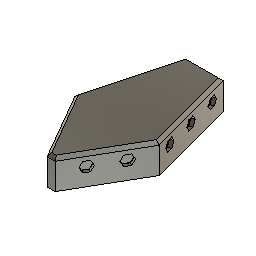
wedge_15deg_2mm (Autodesk Fusion 360 design; units mm, degrees)
Autodesk Fusion 360 part; units mm, degrees
sketch "case_bottom" plane through (0, 0, 0) normal (0, 0, 1) x (1, 0, 0)
  line L0 (-130.2878, -97.5223) -> (-16.5068, -128.0098)
  line L1 (-109.1239, -18.5374) -> (-130.2878, -97.5223)
  line L2 (-16.5068, -128.0098) -> (-3.6943, -109.7118)
  line L3 (-86.9858, -11.6525) -> (-109.1239, -18.5374)
  line L4 (-47.4404, -17.0197) -> (-47.5261, -16.9782)
  line L5 (-47.5261, -16.9782) -> (-66.0896, -12.0041)
  line L6 (-10.9673, -34.7188) -> (-47.4404, -17.0197)
  line L7 (-3.6943, -109.7118) -> (-22.3971, -77.3753)
  line L8 (-22.3971, -77.3753) -> (-10.9673, -34.7188)
  line L9 (-66.0896, -12.0041) -> (-86.9858, -11.6525)
  line L10 (-111.5937, -16.1638) -> (-133.962, -99.6436)
  line L11 (-133.962, -99.6436) -> (-15.2542, -131.4513)
  line L12 (-46.4735, -14.1544) -> (-65.6699, -9.0107)
  line L13 (-65.6699, -9.0107) -> (-87.4169, -8.6449)
  line L14 (-15.2542, -131.4513) -> (-0.1397, -109.8656)
  line L15 (-19.1773, -76.9502) -> (-7.4281, -33.1016)
  line L16 (-0.1397, -109.8656) -> (-19.1773, -76.9502)
  line L17 (-87.4169, -8.6449) -> (-111.5937, -16.1638)
  line L18 (-7.4281, -33.1016) -> (-46.4735, -14.1544)
  line L19 (-65.9217, -10.8067) -> (-87.1583, -10.4495)
  line L20 (-110.1118, -17.588) -> (-131.7575, -98.3709)
  line L21 (-9.5516, -34.0719) -> (-47.1051, -15.8486)
  line L22 (-16.0057, -129.3864) -> (-2.2725, -109.7733)
  line L23 (-47.1051, -15.8486) -> (-65.9217, -10.8067)
  line L24 (-87.1583, -10.4495) -> (-110.1118, -17.588)
  line L25 (-2.2725, -109.7733) -> (-21.1092, -77.2053)
  line L26 (-21.1092, -77.2053) -> (-9.5516, -34.0719)
  line L27 (-131.7575, -98.3709) -> (-16.0057, -129.3864)
  line L28 (-65.8378, -10.208) -> (-87.2445, -9.8479)
  line L29 (-132.4923, -98.7951) -> (-15.7552, -130.0747)
  line L30 (-110.6057, -17.1133) -> (-132.4923, -98.7951)
  line L31 (-46.6545, -15.4003) -> (-46.8946, -15.2839)
  line L32 (-1.5615, -109.8041) -> (-20.4652, -77.1202)
  line L33 (-20.4652, -77.1202) -> (-8.8438, -33.7485)
  line L34 (-15.7552, -130.0747) -> (-1.5615, -109.8041)
  line L35 (-46.8946, -15.2839) -> (-65.8378, -10.208)
  line L36 (-87.2445, -9.8479) -> (-110.6057, -17.1133)
  line L37 (-8.8438, -33.7485) -> (-46.6545, -15.4003)
  circle A0 centre (-88.6378, -32.8795) radius 2.2
  circle A1 centre (-98.4729, -69.5847) radius 2.2
  circle A2 centre (-38.4097, -46.3381) radius 2.2
  circle A3 centre (-34.1664, -92.8451) radius 2.2
  line L38 (-91.0167, -86.1903) -> (-122.8923, -77.6493)
  line L39 (-95.6755, -103.577) -> (-91.0167, -86.1903)
  line L40 (-127.551, -95.0359) -> (-95.6755, -103.577)
  line L41 (-122.8923, -77.6493) -> (-127.551, -95.0359)
  line L42 (-91.5925, -101.9586) -> (-93.1066, -107.6092)
  line L43 (-84.6064, -109.8868) -> (-83.0923, -104.2362)
  line L44 (-83.0923, -104.2362) -> (-91.5925, -101.9586)
  line L45 (-73.6279, -111.4154) -> (-72.7221, -108.0346)
  line L46 (-81.4154, -105.7053) -> (-82.3213, -109.086)
  line L47 (-82.3213, -109.086) -> (-73.6279, -111.4154)
  line L48 (-72.7221, -108.0346) -> (-81.4154, -105.7053)
  line L49 (-12.163, -97.5479) -> (-17.663, -88.0216)
  line L50 (-20.0438, -102.0979) -> (-12.163, -97.5479)
  line L51 (-25.5438, -92.5716) -> (-20.0438, -102.0979)
  line L52 (-17.663, -88.0216) -> (-25.5438, -92.5716)
  line L53 (-96.4921, -72.2377) -> (-98.7956, -80.8345)
  line L54 (-98.7956, -80.8345) -> (-90.4886, -83.0603)
  line L55 (-90.4886, -83.0603) -> (-88.1851, -74.4636)
  line L56 (-88.1851, -74.4636) -> (-96.4921, -72.2377)
  line L57 (1.8603, -131.9251) -> (1.8603, -9.9671)
  line L58 (88.327, -109.8868) -> (86.8129, -104.2362)
  line L59 (137.6826, -99.6436) -> (18.9748, -131.4513)
  line L60 (69.3905, -9.0107) -> (91.1375, -8.6449)
  line L61 (90.7065, -11.6525) -> (112.8445, -18.5374)
  line L62 (90.9651, -9.8479) -> (114.3264, -17.1133)
  line L63 (134.0084, -97.5223) -> (20.2274, -128.0098)
  line L64 (90.8789, -10.4495) -> (113.8324, -17.588)
  line L65 (29.2644, -92.5716) -> (23.7644, -102.0979)
  line L66 (86.8129, -104.2362) -> (95.3131, -101.9586)
  line L67 (21.3836, -88.0216) -> (29.2644, -92.5716)
  line L68 (131.2716, -95.0359) -> (99.3961, -103.577)
  line L69 (50.6152, -15.2839) -> (69.5584, -10.208)
  line L70 (15.8836, -97.5479) -> (21.3836, -88.0216)
  line L71 (91.1375, -8.6449) -> (115.3143, -16.1638)
  line L72 (18.9748, -131.4513) -> (3.8603, -109.8656)
  line L73 (14.6879, -34.7188) -> (51.161, -17.0197)
  line L74 (94.7373, -86.1903) -> (126.6129, -77.6493)
  line L75 (115.3143, -16.1638) -> (137.6826, -99.6436)
  line L76 (5.2822, -109.8041) -> (24.1859, -77.1202)
  line L77 (95.3131, -101.9586) -> (96.8272, -107.6092)
  line L78 (7.4149, -109.7118) -> (26.1177, -77.3753)
  line L79 (99.3961, -103.577) -> (94.7373, -86.1903)
  line L80 (77.3486, -111.4154) -> (76.4427, -108.0346)
  line L81 (69.8103, -12.0041) -> (90.7065, -11.6525)
  line L82 (113.8324, -17.588) -> (135.4781, -98.3709)
  line L83 (19.7263, -129.3864) -> (5.9931, -109.7733)
  line L84 (69.5584, -10.208) -> (90.9651, -9.8479)
  line L85 (91.9058, -74.4636) -> (100.2127, -72.2377)
  line L86 (11.1488, -33.1016) -> (50.1942, -14.1544)
  line L87 (114.3264, -17.1133) -> (136.213, -98.7951)
  line L88 (5.9931, -109.7733) -> (24.8298, -77.2053)
  circle A4 centre (42.1303, -46.3381) radius 2.2
  line L89 (102.5162, -80.8345) -> (94.2092, -83.0603)
  line L90 (85.136, -105.7053) -> (86.0419, -109.086)
  line L91 (69.6424, -10.8067) -> (90.8789, -10.4495)
  line L92 (50.3752, -15.4003) -> (50.6152, -15.2839)
  line L93 (50.1942, -14.1544) -> (69.3905, -9.0107)
  line L94 (22.898, -76.9502) -> (11.1488, -33.1016)
  line L95 (51.161, -17.0197) -> (51.2467, -16.9782)
  line L96 (94.2092, -83.0603) -> (91.9058, -74.4636)
  line L97 (13.2722, -34.0719) -> (50.8257, -15.8486)
  line L98 (112.8445, -18.5374) -> (134.0084, -97.5223)
  line L99 (100.2127, -72.2377) -> (102.5162, -80.8345)
  line L100 (19.4758, -130.0747) -> (5.2822, -109.8041)
  circle A5 centre (102.1935, -69.5847) radius 2.2
  line L101 (50.8257, -15.8486) -> (69.6424, -10.8067)
  circle A6 centre (37.887, -92.8451) radius 2.2
  line L102 (24.1859, -77.1202) -> (12.5644, -33.7485)
  line L103 (24.8298, -77.2053) -> (13.2722, -34.0719)
  line L104 (3.8603, -109.8656) -> (22.898, -76.9502)
  line L105 (136.213, -98.7951) -> (19.4758, -130.0747)
  line L106 (26.1177, -77.3753) -> (14.6879, -34.7188)
  line L107 (135.4781, -98.3709) -> (19.7263, -129.3864)
  line L108 (76.4427, -108.0346) -> (85.136, -105.7053)
  line L109 (12.5644, -33.7485) -> (50.3752, -15.4003)
  line L110 (86.0419, -109.086) -> (77.3486, -111.4154)
  line L111 (51.2467, -16.9782) -> (69.8103, -12.0041)
  line L112 (1.8603, -131.9251) -> (1.8603, -9.9671)
  circle A7 centre (92.3584, -32.8795) radius 2.2
  line L113 (126.6129, -77.6493) -> (131.2716, -95.0359)
  line L114 (23.7644, -102.0979) -> (15.8836, -97.5479)
  line L115 (20.2274, -128.0098) -> (7.4149, -109.7118)
  line L116 (-7.4281, -33.1016) -> (11.1488, -33.1016)
  line L117 (-0.1397, -109.8656) -> (3.8603, -109.8656)
  dimension "d6" = 2
  dimension "d7" = 2
  constraint vertical L57
  constraint horizontal L116
  constraint parallel L116 L117
  measures "d6" distance of L14.end L57
  measures "d7" distance of L72.end L112
extrude "Extrude2" add sketch "case_bottom" along normal blind 14.6 contours L15 L16 L57 L112 L116 L117 | L57 L94 L104 L112 L116 L117
sketch "Sketch3" plane through (1.3449, -0.3604, 0) normal (-0.965926, 0.258819, 0) x (-0.258819, -0.965926, 0)
  line L0 (33.8962, 0) -> (79.2916, 0)
  line L1 (79.2916, 0) -> (79.2916, 14.6)
  line L2 (79.2916, 14.6) -> (33.8962, 14.6)
  line L3 (33.8962, 14.6) -> (33.8962, 0)
  line L4 (33.8962, 8.7) -> (79.2916, 8.7)
  line L5 (43.2082, 6.2181) -> (44.6491, 8.6862)
  line L6 (44.6491, 8.6862) -> (43.2321, 11.1681)
  line L7 (43.2321, 11.1681) -> (40.3743, 11.1819)
  line L8 (40.3743, 11.1819) -> (38.9334, 8.7138)
  line L9 (38.9334, 8.7138) -> (40.3503, 6.2319)
  line L10 (40.3503, 6.2319) -> (43.2082, 6.2181)
  line L11 (55.3561, 6.2286) -> (58.2139, 6.2214)
  line L12 (58.2139, 6.2214) -> (59.6491, 8.6928)
  line L13 (59.6491, 8.6928) -> (58.2264, 11.1714)
  line L14 (58.2264, 11.1714) -> (55.3685, 11.1786)
  line L15 (55.3685, 11.1786) -> (53.9334, 8.7072)
  line L16 (53.9334, 8.7072) -> (55.3561, 6.2286)
  line L17 (70.3545, 6.2295) -> (73.2123, 6.2205)
  line L18 (73.2123, 6.2205) -> (74.6491, 8.6909)
  line L19 (74.6491, 8.6909) -> (73.228, 11.1705)
  line L20 (73.228, 11.1705) -> (70.3701, 11.1795)
  line L21 (70.3701, 11.1795) -> (68.9334, 8.7091)
  line L22 (68.9334, 8.7091) -> (70.3545, 6.2295)
  line L23 (43.3486, 11.3675) -> (40.2598, 11.3824)
  line L24 (40.2598, 11.3824) -> (38.7024, 8.7149)
  line L25 (38.7024, 8.7149) -> (40.2339, 6.0325)
  line L26 (40.2339, 6.0325) -> (43.3227, 6.0176)
  line L27 (43.3227, 6.0176) -> (44.88, 8.6851)
  line L28 (44.88, 8.6851) -> (43.3486, 11.3675)
  line L29 (53.7024, 8.7078) -> (55.2401, 6.0289)
  line L30 (55.2401, 6.0289) -> (58.3289, 6.0211)
  line L31 (58.3289, 6.0211) -> (59.88, 8.6922)
  line L32 (59.88, 8.6922) -> (58.3424, 11.3711)
  line L33 (58.3424, 11.3711) -> (55.2535, 11.3789)
  line L34 (55.2535, 11.3789) -> (53.7024, 8.7078)
  line L35 (70.2384, 6.0299) -> (73.3272, 6.0201)
  line L36 (73.3272, 6.0201) -> (74.88, 8.6902)
  line L37 (74.88, 8.6902) -> (73.3441, 11.3701)
  line L38 (73.3441, 11.3701) -> (70.2553, 11.3799)
  line L39 (70.2553, 11.3799) -> (68.7024, 8.7098)
  line L40 (68.7024, 8.7098) -> (70.2384, 6.0299)
  point P0 (41.7912, 8.7)
  point P1 (56.7912, 8.7)
  point P2 (71.7912, 8.7)
  point P3 (41.7912, 8.7)
  point P4 (56.7912, 8.7)
  point P5 (71.7912, 8.7)
  dimension "d10" = 5.9
  dimension "d11" = 7.895
  dimension "d12" = 15
  dimension "d13" = 15
  dimension "d14" = 2.475
  dimension "d15" = 2.475
  dimension "d16" = 2.475
  dimension "d17" = 0.2
  dimension "d18" = 0.2
  dimension "d19" = 0.2
  constraint coincident L3 L4.start
  constraint coincident L1 L4.end
  constraint perpendicular L1 L4
  constraint coincident L4 P3
  constraint coincident L4 P4
  constraint coincident L4 P5
  constraint coincident P3 P0
  constraint coincident P4 P1
  constraint coincident P5 P2
  measures "d10" distance of L2 L4
  measures "d11" distance of L4.start P3
  measures "d12" distance of P3 P4
  measures "d13" distance of P4 P5
  measures "d14" distance of P3 L10
  measures "d15" distance of P4 L16
  measures "d16" distance of P5 L22
sketch "Sketch4" plane through (2.1265, 0.5698, 0) normal (0.965926, 0.258819, 0) x (-0.258819, 0.965926, 0)
  line L0 (-80.2546, 0) -> (-34.8592, 0)
  line L1 (-34.8592, 0) -> (-34.8592, 14.6)
  line L2 (-34.8592, 14.6) -> (-80.2546, 14.6)
  line L3 (-80.2546, 14.6) -> (-80.2546, 0)
  line L4 (-80.2546, 8.7) -> (-34.8592, 8.7)
  line L5 (-71.3306, 11.1778) -> (-74.1884, 11.1722)
  line L6 (-74.1884, 11.1722) -> (-75.6125, 8.6943)
  line L7 (-75.6125, 8.6943) -> (-74.1786, 6.2222)
  line L8 (-74.1786, 6.2222) -> (-71.3208, 6.2278)
  line L9 (-71.3208, 6.2278) -> (-69.8967, 8.7057)
  line L10 (-69.8967, 8.7057) -> (-71.3306, 11.1778)
  line L11 (-60.6125, 8.7057) -> (-59.1884, 6.2278)
  line L12 (-59.1884, 6.2278) -> (-56.3306, 6.2222)
  line L13 (-56.3306, 6.2222) -> (-54.8967, 8.6943)
  line L14 (-54.8967, 8.6943) -> (-56.3208, 11.1722)
  line L15 (-56.3208, 11.1722) -> (-59.1786, 11.1778)
  line L16 (-59.1786, 11.1778) -> (-60.6125, 8.7057)
  line L17 (-45.6125, 8.7057) -> (-44.1884, 6.2278)
  line L18 (-44.1884, 6.2278) -> (-41.3306, 6.2222)
  line L19 (-41.3306, 6.2222) -> (-39.8967, 8.6943)
  line L20 (-39.8967, 8.6943) -> (-41.3208, 11.1722)
  line L21 (-41.3208, 11.1722) -> (-44.1786, 11.1778)
  line L22 (-44.1786, 11.1778) -> (-45.6125, 8.7057)
  line L23 (-44.3043, 6.0281) -> (-41.2155, 6.0219)
  line L24 (-41.2155, 6.0219) -> (-39.6658, 8.6939)
  line L25 (-39.6658, 8.6939) -> (-41.2049, 11.3719)
  line L26 (-41.2049, 11.3719) -> (-44.2937, 11.3781)
  line L27 (-44.2937, 11.3781) -> (-45.8434, 8.7061)
  line L28 (-45.8434, 8.7061) -> (-44.3043, 6.0281)
  line L29 (-59.3043, 6.0281) -> (-56.2155, 6.0219)
  line L30 (-56.2155, 6.0219) -> (-54.6658, 8.6939)
  line L31 (-54.6658, 8.6939) -> (-56.2049, 11.3719)
  line L32 (-56.2049, 11.3719) -> (-59.2937, 11.3781)
  line L33 (-59.2937, 11.3781) -> (-60.8434, 8.7061)
  line L34 (-60.8434, 8.7061) -> (-59.3043, 6.0281)
  line L35 (-74.3043, 11.3719) -> (-75.8434, 8.6939)
  line L36 (-75.8434, 8.6939) -> (-74.2937, 6.0219)
  line L37 (-74.2937, 6.0219) -> (-71.2049, 6.0281)
  line L38 (-71.2049, 6.0281) -> (-69.6658, 8.7061)
  line L39 (-69.6658, 8.7061) -> (-71.2155, 11.3781)
  line L40 (-71.2155, 11.3781) -> (-74.3043, 11.3719)
  point P0 (-72.7546, 8.7)
  point P1 (-57.7546, 8.7)
  point P2 (-42.7546, 8.7)
  point P3 (-72.7546, 8.7)
  point P4 (-57.7546, 8.7)
  point P5 (-42.7546, 8.7)
  dimension "d20" = 5.9
  dimension "d21" = 7.5
  dimension "d22" = 15
  dimension "d23" = 15
  dimension "d24" = 2.475
  dimension "d25" = 2.475
  dimension "d26" = 2.475
  dimension "d27" = 0.2
  dimension "d28" = 0.2
  dimension "d29" = 0.2
  constraint coincident L3 L4.start
  constraint coincident L1 L4.end
  constraint perpendicular L1 L4
  constraint coincident L4 P3
  constraint coincident L4 P4
  constraint coincident L4 P5
  constraint coincident P3 P0
  constraint coincident P4 P1
  constraint coincident P5 P2
  measures "d20" distance of L2 L4
  measures "d21" distance of L4.start P3
  measures "d22" distance of P3 P4
  measures "d23" distance of P4 P5
  measures "d24" distance of P3 L10
  measures "d25" distance of P4 L16
  measures "d26" distance of P5 L22
sketch "Sketch5" plane through (-47.7203, -27.6005, 0) normal (-0.865639, -0.500669, 0) x (0.500669, -0.865639, 0)
  line L0 (57.0096, 0) -> (95.034, 0)
  line L1 (95.034, 0) -> (95.034, 14.6)
  line L2 (95.034, 14.6) -> (57.0096, 14.6)
  line L3 (57.0096, 14.6) -> (57.0096, 0)
  line L4 (57.0096, 8.7) -> (95.034, 8.7)
  line L5 (69.9359, 11.1765) -> (67.078, 11.1735)
  line L6 (67.078, 11.1735) -> (65.6517, 8.697)
  line L7 (65.6517, 8.697) -> (67.0833, 6.2235)
  line L8 (67.0833, 6.2235) -> (69.9412, 6.2265)
  line L9 (69.9412, 6.2265) -> (71.3675, 8.703)
  line L10 (71.3675, 8.703) -> (69.9359, 11.1765)
  line L11 (80.6517, 8.703) -> (82.078, 6.2265)
  line L12 (82.078, 6.2265) -> (84.9359, 6.2235)
  line L13 (84.9359, 6.2235) -> (86.3675, 8.697)
  line L14 (86.3675, 8.697) -> (84.9412, 11.1735)
  line L15 (84.9412, 11.1735) -> (82.0833, 11.1765)
  line L16 (82.0833, 11.1765) -> (80.6517, 8.703)
  line L17 (66.9623, 11.3734) -> (65.4207, 8.6967)
  line L18 (65.4207, 8.6967) -> (66.968, 6.0234)
  line L19 (66.968, 6.0234) -> (70.0568, 6.0266)
  line L20 (70.0568, 6.0266) -> (71.5984, 8.7033)
  line L21 (71.5984, 8.7033) -> (70.0511, 11.3766)
  line L22 (70.0511, 11.3766) -> (66.9623, 11.3734)
  line L23 (85.0511, 6.0234) -> (86.5984, 8.6967)
  line L24 (86.5984, 8.6967) -> (85.0568, 11.3734)
  line L25 (85.0568, 11.3734) -> (81.968, 11.3766)
  line L26 (81.968, 11.3766) -> (80.4207, 8.7033)
  line L27 (80.4207, 8.7033) -> (81.9623, 6.0266)
  line L28 (81.9623, 6.0266) -> (85.0511, 6.0234)
  point P0 (57.0096, 8.7)
  point P1 (68.5096, 8.7)
  point P2 (83.5096, 8.7)
  point P3 (68.5096, 8.7)
  point P4 (83.5096, 8.7)
  dimension "d30" = 11.5
  dimension "d31" = 15
  dimension "d32" = 2.475
  dimension "d33" = 2.475
  dimension "d34" = 0.2
  dimension "d35" = 0.2
  constraint coincident P0 L4.start
  constraint coincident L1 L4.end
  constraint perpendicular L1 L4
  constraint coincident L4 P3
  constraint coincident L4 P4
  constraint coincident P3 P1
  constraint coincident P4 P2
  measures "d30" distance of P0 P3
  measures "d31" distance of P3 P4
  measures "d32" distance of P3 L10
  measures "d33" distance of P4 L16
sketch "Sketch6" plane through (50.5082, -29.213, 0) normal (0.865639, -0.500669, 0) x (0.500669, 0.865639, 0)
  line L0 (-93.1712, 0) -> (-55.1468, 0)
  line L1 (-55.1468, 0) -> (-55.1468, 14.6)
  line L2 (-55.1468, 14.6) -> (-93.1712, 14.6)
  line L3 (-93.1712, 14.6) -> (-93.1712, 0)
  line L4 (-55.1468, 8.7) -> (-93.1712, 8.7)
  line L5 (-69.5046, 8.6908) -> (-68.0677, 6.2204)
  line L6 (-68.0677, 6.2204) -> (-65.2099, 6.2296)
  line L7 (-65.2099, 6.2296) -> (-63.7889, 8.7092)
  line L8 (-63.7889, 8.7092) -> (-65.2258, 11.1796)
  line L9 (-65.2258, 11.1796) -> (-68.0837, 11.1704)
  line L10 (-68.0837, 11.1704) -> (-69.5046, 8.6908)
  line L11 (-80.2099, 11.1704) -> (-83.0677, 11.1796)
  line L12 (-83.0677, 11.1796) -> (-84.5046, 8.7092)
  line L13 (-84.5046, 8.7092) -> (-83.0837, 6.2296)
  line L14 (-83.0837, 6.2296) -> (-80.2258, 6.2204)
  line L15 (-80.2258, 6.2204) -> (-78.7889, 8.6908)
  line L16 (-78.7889, 8.6908) -> (-80.2099, 11.1704)
  line L17 (-65.0937, 6.03) -> (-63.558, 8.71)
  line L18 (-63.558, 8.71) -> (-65.111, 11.38)
  line L19 (-65.111, 11.38) -> (-68.1998, 11.37)
  line L20 (-68.1998, 11.37) -> (-69.7356, 8.69)
  line L21 (-69.7356, 8.69) -> (-68.1826, 6.02)
  line L22 (-68.1826, 6.02) -> (-65.0937, 6.03)
  line L23 (-80.0937, 11.37) -> (-83.1826, 11.38)
  line L24 (-83.1826, 11.38) -> (-84.7356, 8.71)
  line L25 (-84.7356, 8.71) -> (-83.1998, 6.03)
  line L26 (-83.1998, 6.03) -> (-80.111, 6.02)
  line L27 (-80.111, 6.02) -> (-78.558, 8.69)
  line L28 (-78.558, 8.69) -> (-80.0937, 11.37)
  point P0 (-55.1468, 8.7)
  point P1 (-81.6468, 8.7)
  point P2 (-66.6468, 8.7)
  point P3 (-66.6468, 8.7)
  point P4 (-81.6468, 8.7)
  dimension "d36" = 11.5
  dimension "d37" = 15
  dimension "d38" = 2.475
  dimension "d39" = 2.475
  dimension "d40" = 0.2
  dimension "d41" = 0.2
  constraint coincident P0 L4.start
  constraint coincident L3 L4.end
  constraint perpendicular L3 L4
  constraint coincident L4 P4
  constraint coincident L4 P3
  constraint coincident P3 P2
  constraint coincident P4 P1
  measures "d36" distance of P0 P3
  measures "d37" distance of P4 P3
  measures "d38" distance of P3 L10
  measures "d39" distance of P4 L16
extrude "Extrude3" cut sketch "Sketch6" against normal blind 2 contours L4 L11 L12 L13 L16 | L4 L13 L14 L15 L16 | L4 L5 L6 L7 L10 | L4 L7 L8 L9 L10
extrude "Extrude4" cut sketch "Sketch6" against normal blind 0.2 from surface at -1.8 contours L4 L11 L12 L13 L16 L23 L24 L25 L28 | L4 L13 L14 L15 L16 L25 L26 L27 L28 | L4 L5 L6 L7 L10 L17 L20 L21 L22 | L4 L7 L8 L9 L10 L17 L18 L19 L20
extrude "Extrude5" cut sketch "Sketch5" against normal blind 2 contours L4 L5 L6 L9 L10 | L4 L6 L7 L8 L9 | L4 L11 L12 L13 L14 | L4 L11 L14 L15 L16
extrude "Extrude6" cut sketch "Sketch5" against normal blind 0.2 from surface at -1.8 contours L4 L5 L6 L9 L10 L17 L20 L21 L22 | L4 L6 L7 L8 L9 L17 L18 L19 L20 | L4 L11 L12 L13 L14 L23 L24 L27 L28 | L4 L11 L14 L15 L16 L24 L25 L26 L27
extrude "Extrude7" cut sketch "Sketch3" against normal blind 2 contours L4 L6 L7 L8 L9 | L4 L5 L6 L9 L10 | L4 L17 L18 L19 L22 | L4 L19 L20 L21 L22 | L4 L13 L14 L15 L16 | L4 L11 L12 L13 L16
extrude "Extrude8" cut sketch "Sketch3" against normal blind 0.2 from surface at -1.8 contours L4 L6 L7 L8 L9 L23 L24 L25 L28 | L4 L5 L6 L9 L10 L25 L26 L27 L28 | L4 L17 L18 L19 L22 L35 L36 L37 L40 | L4 L19 L20 L21 L22 L37 L38 L39 L40 | L4 L13 L14 L15 L16 L29 L32 L33 L34 | L4 L11 L12 L13 L16 L29 L30 L31 L32
extrude "Extrude9" cut sketch "Sketch4" against normal blind 2 contours L4 L5 L6 L9 L10 | L4 L6 L7 L8 L9 | L4 L17 L18 L19 L20 | L4 L17 L20 L21 L22 | L4 L11 L14 L15 L16 | L4 L11 L12 L13 L14
extrude "Extrude10" cut sketch "Sketch4" against normal blind 0.2 from surface at -1.8 contours L4 L5 L6 L9 L10 L35 L38 L39 L40 | L4 L6 L7 L8 L9 L35 L36 L37 L38 | L4 L17 L18 L19 L20 L23 L24 L25 L28 | L4 L17 L20 L21 L22 L25 L26 L27 L28 | L4 L11 L14 L15 L16 L31 L32 L33 L34 | L4 L11 L12 L13 L14 L29 L30 L31 L34
chamfer "Chamfer1" distance 1.5 angle 45 6 edges at (13.3791, -93.4079, 14.6) (17.0234, -55.0259, 14.6) (1.8603, -33.1016, 14.6) (-13.3027, -55.0259, 14.6) (-9.6585, -93.4079, 14.6) (1.8603, -109.8656, 14.6)
equation "rotation = 15 deg"
equation "mirror_offset = 2 mm"
equation "d6 = mirror_offset"
equation "d7 = mirror_offset"
